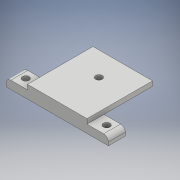
# Autodesk Inventor part: Enclosure clip simple
Saved by Autodesk Inventor 2018 (Build 220112000, 112)
## iProperties
Created: 2018-03-29
Part Number: Enclosure clip simple
Material: Generic
Document SubType Name: Modeling
Designer: elect
Density: 1 g/cm^3
Appearance: Default
Author: elect
Autodesk Inventor part; units mm, degrees
ref_plane "YZ Plane" through (0, 0, 0) normal (1, 0, 0) x (0, 1, 0)
ref_plane "XZ Plane" through (0, 0, 0) normal (0, 1, 0) x (-1, 0, 0)
ref_plane "XY Plane" through (0, 0, 0) normal (0, 0, 1) x (1, 0, 0)
sketch "Sketch1" plane through (0, 0, 0) normal (0, 0, 1) x (1, 0, 0)
  line L0 (0, 0) -> (-43, 0)
  line L1 (-43, 0) -> (-43, -7.5)
  line L2 (-43, -7.5) -> (0, -7.5)
  line L3 (0, -7.5) -> (0, 0)
  dimension "d0" = 43
  dimension "d1" = 7.5
  constraints: 8 end point, 2 parallel, 1 horizontal, 1 perpendicular
  measures "d0" distance of L2.end L1.end
  measures "d1" distance of L1.end L0.end
extrude "Extrusion1" add sketch "Sketch1" along normal blind 3.4
sketch "Sketch3" plane through (0, 0, 3.4) normal (0, 0, 1) x (1, 0, 0)
  circle A0 centre (-38.5, -3.75) radius 1.5
  circle A1 centre (-4.5, -3.75) radius 1.5
  point P0 (0, 0)
  dimension "d4" = 3
  dimension "d5" = 3
  constraints: 2 centre point
  measures "d4" diameter of A0
  measures "d5" diameter of A1
hole "Hole1" at (-38.5, -3.75, 3.4) at (-4.5, -3.75, 3.4) direction (0, 0, -1) diameter 2.8 end through all
sketch "Sketch4" plane through (0, 0, 3.4) normal (0, 0, 1) x (1, 0, 0)
  line L0 (-43, 0) -> (-43, -7.5) projected
  line L1 (-43, 0) -> (-34, 0)
  line L2 (-34, 0) -> (-34, -3.75)
  line L3 (-34, -3.75) -> (-43, -3.75)
  line L4 (-43, -3.75) -> (-43, 0)
  line L5 (0, 0) -> (-9, 0)
  line L6 (-9, 0) -> (-9, -3.75)
  line L7 (-9, -3.75) -> (0, -3.75)
  line L8 (0, -3.75) -> (0, 0)
  line L9 (-9, 0) -> (-34, 0)
  line L10 (-34, 0) -> (-34, -2)
  line L11 (-34, -2) -> (-9, -2)
  line L12 (-9, -2) -> (-9, 0)
  dimension "d13" = 9
  dimension "d14" = 9
  dimension "d15" = 2
  constraints: 24 end point, 6 parallel, 3 horizontal, 3 perpendicular, 2 point on line
  measures "d13" distance of L2.end L3.end
  measures "d14" distance of L7.end L6.end
  measures "d15" distance of L10.end L9.end
extrude "Extrusion2" add sketch "Sketch4" along normal blind 2 contours L9 L6 L11 L2
sketch "Sketch5" plane through (-43, 0, 0) normal (0, 1, 0) x (1, 0, 0)
  line L0 (43, -3.4) -> (34, -3.4) projected
  line L1 (9, -5.4) -> (34, -5.4) projected
  line L2 (34, -3.4) -> (9, -3.4)
  line L3 (9, -3.4) -> (9, -5.4)
  line L4 (9, -5.4) -> (34, -5.4)
  line L5 (34, -5.4) -> (34, -3.4)
  point P0 (43, 0)
  constraints: 8 end point, 2 parallel, 1 horizontal, 1 perpendicular
extrude "Extrusion3" add sketch "Sketch5" along normal blind 20 and the other way blind 7.5
sketch "Sketch6" plane through (-43, 0, 0) normal (0, 1, 0) x (1, 0, 0)
  line L0 (43, 0) -> (43, -3.4) projected
  line L1 (0, 0) -> (0, -3.4) projected
  line L2 (43, 0) -> (0, 0)
  line L3 (0, 0) -> (0, -3.4)
  line L4 (0, -3.4) -> (43, -3.4)
  line L5 (43, -3.4) -> (43, 0)
  dimension "d22" = 43
  constraints: 8 end point, 2 parallel, 1 horizontal, 1 perpendicular
  measures "d22" distance of L4.end L1.end
extrude "Extrusion4" cut sketch "Sketch6" against normal blind 0.4
fillet "Fillet3" radius 2 1 edges at (-43, -3.95, 3.4)
fillet "Fillet4" radius 2 1 edges at (0, -3.95, 3.4)
sketch "Sketch7" plane through (0, 0, 5.4) normal (0, 0, 1) x (1, 0, 0)
  line L0 (-9, -7.5) -> (-34, -7.5) projected
  line L1 (-9, -7.5) -> (-21.5, -7.5)
  line L2 (-21.5, -7.5) -> (-21.5, 0)
  line L3 (-21.5, 0) -> (-9, 0)
  line L4 (-9, 0) -> (-9, -7.5)
  line L5 (-21.5, 0) -> (-21.5, 10)
  circle A0 centre (-21.5, 10) radius 1.4
  point P0 (0, 0)
  dimension "d32" = 12.5
  dimension "d33" = 7.5
  dimension "d34" = 10
  dimension "d35" = 2.8
  constraints: 10 end point, 2 parallel, 1 centre point, 1 coincident, 1 horizontal, 1 perpendicular, 1 vertical
  measures "d32" distance of L2.end L3.end
  measures "d33" distance of L1.end L2.end
  measures "d34" distance of L2.end L5.end
  measures "d35" diameter of A0
hole "Hole2" at (-21.5, 10, 5.4) direction (0, 0, -1) diameter 2.8 end through all
body "Solid1"
